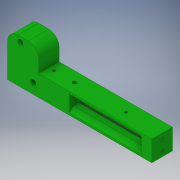
# Autodesk Inventor part: BackTopBeams
Saved by Autodesk Inventor 2019 (Build 230136000, 136)
## iProperties
Created: 2019-10-01
Part Number: BackTopBeams
Material: Generic
Document SubType Name: Modeling
Designer: james
Density: 1 g/cm^3
Appearance: Dark Green
Mass: 163.351 g
Surface Area: 274.632 cm^2
Volume: 163.351 cm^3
Author: james
Autodesk Inventor part; units mm, degrees
ref_plane "YZ Plane" through (0, 0, 0) normal (1, 0, 0) x (0, 1, 0)
ref_plane "XZ Plane" through (0, 0, 0) normal (0, 1, 0) x (-1, 0, 0)
ref_plane "XY Plane" through (0, 0, 0) normal (0, 0, 1) x (1, 0, 0)
sketch "Sketch1" plane through (0, 0, 0) normal (1, 0, 0) x (0, 1, 0)
  line L0 (12.3116, 18.9917) -> (-13.0884, 18.9917)
  line L1 (-13.0884, 18.9917) -> (-13.0884, -6.4083)
  line L2 (-13.0884, -6.4083) -> (12.3116, -6.4083)
  line L3 (12.3116, -6.4083) -> (12.3116, 18.9917)
  point P0 (0, 0)
  dimension "d0" = 25.4
  dimension "d1" = 25.4
  constraints: 8 end point, 2 parallel, 1 horizontal, 1 perpendicular
  measures "d0" distance of L1.end L2.end
  measures "d1" distance of L2.end L0.start
extrude "Extrusion1" add sketch "Sketch1" along normal blind 177.8
sketch "Sketch5" plane through (177.8, 0, 0) normal (1, 0, 0) x (0, 0, -1)
  line L0 (-18.9917, -13.0884) -> (6.4083, -13.0884) projected
  line L1 (-18.9917, 12.3116) -> (-18.9917, -13.0884) projected
  point P0 (0, 0)
  point P1 (-6.2917, 5.9616)
  point P2 (-6.2917, -6.7384)
  dimension "d31" = 6.35
  dimension "d32" = 19.05
  dimension "d33" = 12.7
  dimension "d34" = 12.7
  measures "d31" distance from line of L0 point (-6.292, -6.738)
  measures "d32" distance from line of point (-6.292, 5.962) L0
  measures "d33" distance from line of L1 point (-6.292, 5.962)
  measures "d34" distance from line of L1 point (-6.292, -6.738)
hole "Hole4" at (177.8, 5.9616, 6.2917) at (177.8, -6.7384, 6.2917) direction (-1, 0, 0) diameter 3.302 end through all thread size "8-32 UNC" class "2B" standard "ANSI Unified Screw Threads"
sketch "Sketch8" plane through (0, 12.3116, 18.9917) normal (0, 1, 0) x (1, 0, 0)
  line L0 (0, 25.4) -> (38.1, 25.4)
  line L1 (38.1, 25.4) -> (38.1, 0)
  line L2 (38.1, 0) -> (0, 0)
  line L3 (0, 0) -> (0, 25.4)
  line L4 (0, 25.4) -> (0, 0) projected
  line L5 (0, 25.4) -> (177.8, 25.4) projected
  line L6 (0, 0) -> (177.8, 0) projected
  point P0 (0, 18.9917)
  dimension "d60" = 0
  dimension "d61" = 38.1
  dimension "d62" = 0
  dimension "d63" = 0
  constraints: 8 end point, 2 parallel, 1 horizontal, 1 perpendicular
  measures "d60" distance between parallel lines of L4 L3
  measures "d61" distance of L0.start L0.end
  measures "d62" distance between parallel lines of L5 L0
  measures "d63" distance between parallel lines of L2 L6
extrude "Extrusion2" add sketch "Sketch8" along normal blind 28.575
fillet "Fillet1" radius 12.7 2 edges at (38.1, 40.8866, 6.2917) (0, 40.8866, 6.2917)
sketch "Sketch9" plane through (0, -13.0884, 18.9917) normal (0, 0, 1) x (1, 0, 0)
  line L0 (0, 41.275) -> (0, 0) projected
  line L1 (12.7, 53.975) -> (25.4, 53.975) projected
  line L2 (38.1, 25.4) -> (177.8, 25.4) projected
  point P0 (0, 13.0884)
  point P1 (15.875, 47.625)
  dimension "d67" = 15.875
  dimension "d137" = 22.225
  measures "d67" distance from line of L0 point (15.875, 47.625)
  measures "d137" distance from line of point (15.875, 47.625) L2
hole "Hole7" at (15.875, 34.5366, 18.9917) direction (0, 0, -1) diameter 6.477 end through all
sketch "Sketch10" plane through (0, -13.0884, 18.9917) normal (0, 0, 1) x (1, 0, 0)
  line L0 (0, 0) -> (177.8, 0) projected
  line L1 (0, 41.275) -> (0, 0) projected
  point P0 (0, 13.0884)
  point P1 (31.75, 12.7)
  dimension "d76" = 12.7
  dimension "d77" = 31.75
  measures "d76" distance from line of L0 point (31.75, 12.7)
  measures "d77" distance from line of L1 point (31.75, 12.7)
hole "Hole8" at (31.75, -0.3884, 18.9917) direction (0, 0, -1) diameter 6.477 end through all
sketch "Sketch11" plane through (177.8, 12.3116, 18.9917) normal (0, 1, 0) x (1, 0, 0)
  line L0 (-177.8, 25.4) -> (-177.8, 0) projected
  line L1 (-139.7, 0) -> (0, 0) projected
  point P0 (-177.8, 18.9917)
  point P1 (-107.95, 12.7)
  dimension "d85" = 69.85
  dimension "d86" = 12.7
  measures "d85" distance from line of point (-107.95, 12.7) L0
  measures "d86" distance from line of L1 point (-107.95, 12.7)
hole "Hole9" at (69.85, 12.3116, 6.2917) direction (0, -1, 0) diameter 4.4958 end through all clearance for "Flat Head Machine Screw (82)" size "#8" standard "Ansi Unified Screw Threads"
sketch "Sketch12" plane through (177.8, 0, 0) normal (1, 0, 0) x (0, 0, -1)
  line L0 (-18.9917, 9.7716) -> (-18.9917, -10.5484)
  line L1 (-18.9917, -10.5484) -> (-13.9117, -5.4684)
  line L2 (-13.9117, -5.4684) -> (1.3283, -5.4684)
  line L3 (1.3283, -5.4684) -> (6.4083, -10.5484)
  line L4 (6.4083, -10.5484) -> (6.4083, 9.7716)
  line L5 (6.4083, 9.7716) -> (1.3283, 4.6916)
  line L6 (1.3283, 4.6916) -> (-13.9117, 4.6916)
  line L7 (-13.9117, 4.6916) -> (-18.9917, 9.7716)
  line L8 (-18.9917, 12.3116) -> (-18.9917, -13.0884) projected
  line L9 (-18.9917, -13.0884) -> (6.4083, -13.0884) projected
  dimension "d103" = 20.32
  dimension "d104" = 5.08
  dimension "d105" = 5.08
  dimension "d106" = 5.08
  dimension "d107" = 25.4
  dimension "d108" = 5.08
  dimension "d109" = 0
  dimension "d110" = 0
  dimension "d111" = 0
  dimension "d112" = 2.54
  constraints: 16 end point, 3 perpendicular, 2 parallel, 1 vertical
  measures "d103" distance of L0.start L0.end
  measures "d104" distance from line of L0.start L6
  measures "d105" distance from line of L0.end L2
  measures "d106" distance from line of L6 L4.end
  measures "d107" distance between parallel lines of L0 L4
  measures "d108" distance from line of L2 L3.end
  measures "d109" horizontal distance of L5.end L2.end
  measures "d110" horizontal distance of L1.end L6.end
  measures "d111" distance between parallel lines of L0 L8
  measures "d112" distance from line of L9 L0.end
extrude "Extrusion3" cut sketch "Sketch12" against normal blind 101.6
sketch "Sketch13" plane through (177.8, 0, 0) normal (1, 0, 0) x (0, 0, -1)
  line L0 (-18.9917, 12.3116) -> (6.4083, 12.3116)
  line L1 (6.4083, 12.3116) -> (6.4083, -13.0884)
  line L2 (6.4083, -13.0884) -> (-18.9917, -13.0884)
  line L3 (-18.9917, -13.0884) -> (-18.9917, 12.3116)
  line L4 (6.4083, 9.7716) -> (6.4083, -10.5484) projected
  line L5 (-18.9917, -13.0884) -> (6.4083, -13.0884) projected
  point P0 (0, 0)
  dimension "d115" = 25.4
  dimension "d116" = 25.4
  dimension "d117" = 0
  dimension "d118" = 0
  constraints: 8 end point, 2 parallel, 1 horizontal, 1 perpendicular
  measures "d115" distance of L1.end L2.end
  measures "d116" distance of L0.end L1.end
  measures "d117" distance between parallel lines of L4 L1
  measures "d118" distance between parallel lines of L5 L2
extrude "Extrusion4" add sketch "Sketch13" against normal blind 12.7
sketch "Sketch14" plane through (177.8, 0, 0) normal (1, 0, 0) x (0, 0, -1)
  arc A0 (-5.2368, 4.6916) -> (-7.3467, 4.6916) centre (-6.2917, 5.9616) ccw projected
  arc A1 (-7.3467, -5.4684) -> (-5.2368, -5.4684) centre (-6.2917, -6.7384) ccw projected
  point P0 (0, 0)
  constraints: 2 coincident
hole "Hole10" at (177.8, 5.9616, 6.2917) at (177.8, -6.7384, 6.2917) direction (-1, 0, 0) diameter 3.302 end through all thread size "8-32 UNC" class "2B" standard "ANSI Unified Screw Threads"
sketch "Sketch15" plane through (177.8, 12.3116, 18.9917) normal (0, 1, 0) x (1, 0, 0)
  line L0 (-139.7, 25.4) -> (0, 25.4) projected
  line L1 (-139.7, 0) -> (-139.7, 25.4) projected
  point P0 (-177.8, 18.9917)
  point P1 (-133.35, 12.7)
  dimension "d128" = 12.7
  dimension "d129" = 6.35
  measures "d128" distance from line of L0 point (-133.35, 12.7)
  measures "d129" distance from line of L1 point (-133.35, 12.7)
hole "Hole11" at (44.45, 12.3116, 6.2917) direction (0, -1, 0) diameter 3.302 end through all thread size "8-32 UNC" class "2B" standard "ANSI Unified Screw Threads"
sketch "Sketch16" plane through (177.8, 12.3116, 18.9917) normal (0, 1, 0) x (1, 0, 0)
  line L0 (-12.7, 20.32) -> (-101.6, 20.32) projected
  circle A0 centre (-107.95, 12.7) radius 2.2479 projected
  line L1 (-139.7, 0) -> (0, 0) projected
  point P0 (-177.8, 18.9917)
  point P1 (-44.45, 12.7)
  dimension "d138" = 63.5
  dimension "d139" = 12.7
  measures "d138" distance of point (-44.45, 12.7) A0.centre
  measures "d139" distance from line of L1 point (-44.45, 12.7)
hole "Hole12" at (133.35, 12.3116, 6.2917) direction (0, -1, 0) diameter 3.302 depth 12.2936 tip angle 118.188 thread size "8-32 UNC" class "2B" standard "ANSI Unified Screw Threads"
body "Solid1"
